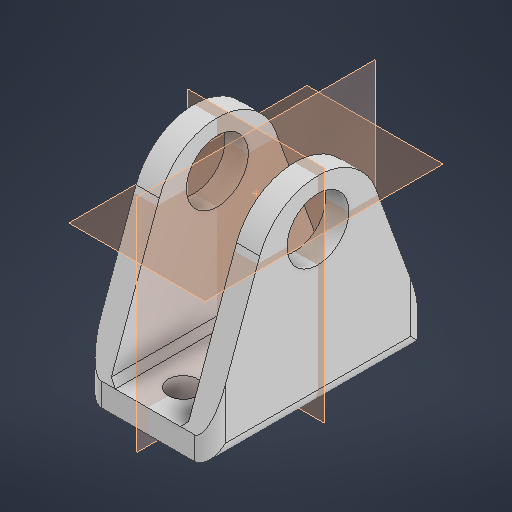
# Autodesk Inventor part: 0.5 in Rod End Bracket (Rough)
Saved by Autodesk Inventor 2026.1 (Build 301233000, 233)
## iProperties
Created: 2026-06-16
Part Number: 0.5 in Rod End Bracket (Rough)
Material: Generic
Document SubType Name: Sheet Metal
Designer: share
Density: 1 g/cm^3
Sheet Metal Rule: Default
Appearance: Default
Author: share
Autodesk Inventor part; units mm, degrees
sketch "Sketch1" plane through (0, 0, 0) normal (0, 1, 0) x (-1, 0, 0)
  line L0 (7.9375, 22.225) -> (-7.9375, 22.225)
  line L1 (-7.9375, 22.225) -> (-7.9375, -22.225)
  line L2 (-7.9375, -22.225) -> (7.9375, -22.225)
  line L3 (7.9375, -22.225) -> (7.9375, 22.225)
  line L4 (7.9375, 22.225) -> (-7.9375, -22.225) construction
  line L5 (-7.9375, 22.225) -> (7.9375, -22.225) construction
  point P0 (0, 0)
  point P1 (-50.8, 0)
  dimension "d0" = 15.875
  dimension "d1" = 44.45
  constraints: 12 end point, 2 midpoint, 2 parallel, 1 horizontal, 1 perpendicular
  measures "d0" distance between parallel lines of L1 L3
  measures "d1" distance between parallel lines of L2 L0
extrude "Base" add sketch "Sketch1" along normal blind 4.7625
sketch "Sketch2" plane through (7.9375, 0, 22.225) normal (1, 0, 0) x (0, 0, -1)
  line L0 (0, 0) -> (0, 4.7625) projected
  line L1 (0, 4.7625) -> (10.2968, 32.9347)
  line L2 (0, 4.7625) -> (44.45, 4.7625) projected
  line L3 (34.1532, 32.9347) -> (44.45, 4.7625)
  line L4 (0, 0) -> (44.45, 0) projected
  arc A0 (34.1532, 32.9347) -> (10.2968, 32.9347) centre (22.225, 28.575) ccw
  line L5 (0, 0) -> (44.45, 0) projected
  line L6 (44.45, 0) -> (44.45, 4.7625) projected
  line L7 (0, 4.7625) -> (44.45, 4.7625) projected
  line L8 (0, 0) -> (0, 4.7625) projected
  point P0 (22.225, 0)
  point P1 (22.225, 41.275)
  dimension "d10" = 12.7
  dimension "d12" = 41.275
  constraints: 4 end point, 3 point on circle, 2 tangent, 1 centre point, 1 equal length
  measures "d10" radius of A0
  measures "d12" distance from line of L4 point (22.225, 41.275)
extrude "Vertical 1" add sketch "Sketch2" along normal blind 4.7625
sketch "Sketch5" plane through (-7.9375, 0, -22.225) normal (-1, 0, 0) x (0, 0, 1)
  line L0 (44.45, 4.7625) -> (44.45, 0) projected
  line L1 (44.45, 0) -> (0, 0) projected
  line L2 (0, 0) -> (0, 4.7625) projected
  line L3 (0, 4.7625) -> (10.2968, 32.9347) projected
  arc A0 (34.1532, 32.9347) -> (10.2968, 32.9347) centre (22.225, 28.575) ccw projected
  line L4 (34.1532, 32.9347) -> (44.45, 4.7625) projected
extrude "Vertical 2" add sketch "Sketch5" along normal blind 4.7625
sketch "Sketch6" plane through (12.7, 0, 22.225) normal (1, 0, 0) x (0, 0, -1)
  line L0 (22.225, 0) -> (22.225, 41.275) construction
  arc A0 (34.1532, 32.9347) -> (10.2968, 32.9347) centre (22.225, 28.575) ccw projected
  circle A1 centre (22.225, 31.75) radius 6.35
  dimension "d29" = 12.7
  dimension "d30" = 9.525
  constraints: 2 end point, 2 point on circle, 1 centre point, 1 point on line, 1 vertical
  measures "d29" diameter of A1
  measures "d30" distance of A1.centre point (22.225, 41.275)
extrude "Extrusion8" cut sketch "Sketch6" against normal through all
fillet "Fillet2" radius 3.175 6 edges at (-12.7, 0, 0) (-12.7, 2.3813, -22.225) (12.7, 2.3813, -22.225) (12.7, 2.3813, 22.225) (12.7, 0, 0) (-12.7, 2.3813, 22.225)
chamfer "Chamfer2" distance 1.27 angle 45 2 edges at (-7.9375, 4.7625, 0) (7.9375, 4.7625, 0)
ref_plane "Work Plane2" through (0, 31.75, 0) normal (0, 1, 0) x (-1, 0, 0)
sketch "Sketch7" plane through (0, 4.7625, 0) normal (0, 1, 0) x (1, 0, 0)
  line L0 (0, 31.115) -> (0, -31.115) construction
  line L1 (17.78, 0) -> (-17.78, 0) construction
  point P0 (0, 0)
  point P1 (0, -15)
  point P2 (0, 15)
  dimension "d37" = 30
  constraints: 2 point on line, 1 symmetric about line
  measures "d37" distance of point (0, 15) point (0, -15)
hole "Hole1" at (0, 4.7625, 15) at (0, 4.7625, -15) direction (0, -1, 0) diameter 6 end through all
ref_plane "Work Plane1" through (0, 0, 22.225) normal (-1, 0, 0) x (0, 0, 1)
equation "\"d43\" = Thickness"
equation "\"BendRadius\" = Thickness"
equation "\"BendReliefWidth\" = Thickness"
equation "\"BendReliefDepth\" = 0.5 * Thickness"
equation "\"CornerReliefSize\" = 4 * Thickness"
equation "\"MinimumRemnant\" = 2 * Thickness"
equation "\"TransitionRadius\" = BendRadius"
equation "\"JacobiRadiusSize\" = BendRadius"
equation "\"GapSize\" = Thickness"
equation "\"Thickness\" = 3.048"
body "Solid2"
